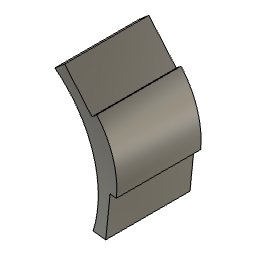
corner_frontmost v1 (Autodesk Fusion 360 design; units mm, degrees)
Autodesk Fusion 360 part; units mm, degrees
sketch "Front Most Corner" plane through (0, 0, 0) normal (0, 1, 0) x (1, 0, 0)
  circle A0 centre (2048.0968, -93.3767) radius 25 construction
  line L0 (1842.0683, -371.981) -> (2073.5797, -102.0665)
  line L1 (2073.9927, -100.7451) -> (2060.9213, 25.5804)
  line L2 (2072.964, -90.8036) -> (2048.0968, -93.3767) construction
  line L3 (2072.964, -90.8036) -> (2071.0691, -90.9997)
  line L4 (2071.0691, -90.9997) -> (2069.762, -78.3671)
  line L5 (2069.762, -78.3671) -> (2065.9722, -78.7593)
  line L6 (2067.0728, -109.6528) -> (2065.6268, -108.4126)
  line L7 (2065.6268, -108.4126) -> (2057.3585, -118.0524)
  arc A1 (2067.0728, -109.6528) -> (2072.964, -90.8036) centre (2048.0968, -93.3767) ccw
  line L8 (2057.3585, -118.0524) -> (2054.4666, -115.5719)
  line L9 (2048.0968, -93.3767) -> (2071.9585, -100.8346) construction
  arc A2 (2054.4666, -115.5719) -> (2065.9722, -78.7593) centre (2033.7666, -88.8979) ccw
  point P0 (2065.993, -98.9701)
  dimension "d1" = 50
  dimension "d2" = 25
  dimension "d3" = 25
  measures "d1" diameter of A0
  measures "d2" distance of L9.end A0.centre
  measures "d3" distance of L2.start A0.centre
extrude "Extrude1" add sketch "Front Most Corner" along normal blind 25.4
